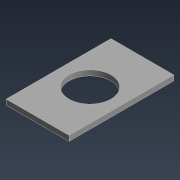
# Autodesk Inventor part: P017-Carter_chapeau
Saved by Autodesk Inventor 2021.3 (Build 253353000, 353)
## iProperties
Created: 2022-04-01
Part Number: P017-Carter_chapeau
Material: Générique
Document SubType Name: Modeling
Designer: remi
Density: 1 g/cm^3
Appearance: Par défaut
Author: remi
Autodesk Inventor part; units mm, degrees
ref_plane "YZ Plane" through (0, 0, 0) normal (1, 0, 0) x (0, 1, 0)
ref_plane "XZ Plane" through (0, 0, 0) normal (0, 1, 0) x (-1, 0, 0)
ref_plane "XY Plane" through (0, 0, 0) normal (0, 0, 1) x (1, 0, 0)
sketch "Sketch2" plane through (0, 0, 0) normal (0, 0, 1) x (1, 0, 0)
  line L0 (-30, -50) -> (30, -50)
  line L1 (30, -50) -> (30, 50)
  line L2 (30, 50) -> (-30, 50)
  line L3 (-30, 50) -> (-30, -50)
  line L4 (-30, -50) -> (30, 50) construction
  line L5 (30, -50) -> (-30, 50) construction
  point P0 (0, 0)
  dimension "d0" = 60
  dimension "d1" = 100
  constraints: 12 end point, 2 midpoint, 2 parallel, 1 horizontal, 1 perpendicular
  measures "d0" distance of L1.end L2.end
  measures "d1" distance of L0.end L1.end
extrude "Extrusion1" add sketch "Sketch2" along normal blind 5
sketch "Sketch3" plane through (0, 0, 5) normal (0, 0, 1) x (1, 0, 0)
  circle A0 centre (0, 0) radius 20
  line L0 (-30, 50) -> (-30, -50) construction
  line L1 (30, -50) -> (30, 50) construction
  line L2 (30, 50) -> (-30, 50) construction
  line L3 (-30, 50) -> (-30, -50) construction
  line L4 (-30, -50) -> (30, -50) construction
  dimension "d5" = 60
  dimension "d6" = 40
  constraints: 1 centre point, 1 coincident
  measures "d5" distance of L1.end L2.end
  measures "d6" diameter of A0
extrude "Extrusion2" cut sketch "Sketch3" against normal blind 5
body "Solid1"
